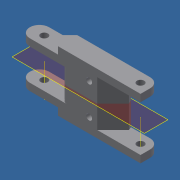
# Autodesk Inventor part: FingerPartA
Saved by Autodesk Inventor 2014 SP2 (Build 180246200, 246)
## iProperties
Created: 2014-12-28
Part Number: FingerPartA
Material: Generisch
Document SubType Name: Modeling
Designer: 4ndreas
Density: 1 g/cm^3
Appearance: Vorgabe
Mass: 4.96399 g
Surface Area: 30.3488 cm^2
Volume: 4.96399 cm^3
Author: 4ndreas
Autodesk Inventor part; units mm, degrees
ref_plane "YZ Plane" through (0, 0, 0) normal (1, 0, 0) x (0, 1, 0)
ref_plane "XZ Plane" through (0, 0, 0) normal (0, 1, 0) x (-1, 0, 0)
ref_plane "XY Plane" through (0, 0, 0) normal (0, 0, 1) x (1, 0, 0)
sketch "Skizze1" plane through (0, 0, 0) normal (0, 0, 1) x (1, 0, 0)
  circle A0 centre (0, 0) radius 4 construction
  circle A1 centre (40, 0) radius 4 construction
  line L0 (0, 0) -> (40, 0) construction
  arc A2 (0, 4) -> (0, -4) centre (0, 0) ccw
  arc A3 (44, 0) -> (40, 4) centre (40, 0) ccw
  line L1 (0, 4) -> (40, 4)
  line L2 (0, -4) -> (44, -4)
  line L3 (44, -4) -> (44, 0)
  dimension "d0" = 8
  dimension "d1" = 40
  constraints: 8 end point, 6 tangent, 4 centre point, 4 point on circle, 2 coincident, 1 equal radius, 1 horizontal, 1 parallel, 1 perpendicular
  measures "d0" diameter of A0
  measures "d1" distance of L0.start L0.end
extrude "Extrusion1" add sketch "Skizze1" along normal blind 3
sketch "Skizze2" plane through (0, 0, 3) normal (0, 0, 1) x (1, 0, 0)
  arc A0 (0, 4) -> (0, -4) centre (0, 0) ccw projected
  line L0 (0, -4) -> (44, -4) projected
  line L1 (44, -4) -> (44, 0) projected
  arc A1 (44, 0) -> (40, 4) centre (40, 0) ccw projected
  line L2 (40, 4) -> (0, 4) projected
  line L3 (6, 4) -> (34, 4)
  line L4 (34, 4) -> (34, -4)
  line L5 (34, -4) -> (6, -4)
  line L6 (6, -4) -> (6, 4)
  line L7 (0, 0) -> (-4, 0) construction
  line L8 (-4, 0) -> (-4, -4) construction
  line L9 (-4, -4) -> (0, -4) construction
  line L10 (0, -4) -> (0, 0) construction
  dimension "d4" = 10
  dimension "d5" = 4
  dimension "d6" = 10
  constraints: 16 end point, 4 parallel, 2 horizontal, 2 perpendicular, 2 point on line, 2 tangent
  measures "d4" distance between parallel lines of L4 L1
  measures "d5" radius of A1
  measures "d6" distance between parallel lines of L8 L6
extrude "Extrusion2" add sketch "Skizze2" along normal blind 9.5 contours L2 L4 L0 L6
sketch "Skizze3" plane through (0, 0, 0) normal (0, 0, -1) x (-1, 0, 0)
  line L0 (-6, -4) -> (-6, 4) projected
  line L1 (-6, 4) -> (0, 4) projected
  arc A0 (0, -4) -> (0, 4) centre (0, 0) ccw projected
  line L2 (0, -4) -> (-6, -4) projected
sketch "Skizze4" plane through (0, 0, 3) normal (0, 0, 1) x (1, 0, 0)
  line L0 (6, -4) -> (6, 4) projected
  line L1 (6, 4) -> (0, 4) projected
  arc A0 (0, 4) -> (0, -4) centre (0, 0) ccw projected
  line L2 (0, -4) -> (6, -4) projected
extrude "Extrusion3" add sketch "Skizze4" along normal blind 3
extrude "Extrusion4" cut sketch "Skizze3" against normal blind 3
sketch "Skizze5" plane through (0, 0, 0) normal (0, 0, -1) x (-1, 0, 0)
  line L0 (-6, -4) -> (-6, 4) projected
  line L1 (-40, 4) -> (-6, 4) projected
  arc A0 (-40, 4) -> (-44, 0) centre (-40, 0) ccw projected
  line L2 (-6, -4) -> (-44, -4) projected
  line L3 (-6, 0.3) -> (-9.7, 4)
  line L4 (-9.7, -4) -> (-6, -0.3)
  line L5 (-9.7, 4) -> (-6, 4)
  line L6 (-6, 0.3) -> (-6, 4)
  line L7 (0, 0) -> (-40, 0) construction
  circle A1 centre (0, 0) radius 4
  line L8 (-6, -4) -> (-6, 4) projected
  line L9 (0, -4) -> (-6, -4) projected
  arc A2 (0, -4) -> (0, 4) centre (0, 0) ccw projected
  line L10 (-6, 4) -> (0, 4) projected
  line L11 (-3.0018, 2.6437) -> (3.0018, -2.6437)
  line L12 (3.0018, -2.6437) -> (-9.9619, -17.3635)
  line L13 (-9.9619, -17.3635) -> (-15.9655, -12.0761)
  line L14 (-15.9655, -12.0761) -> (-3.0018, 2.6437)
  dimension "d13" = 45
  dimension "d14" = 0.6
  constraints: 18 end point, 6 point on line, 2 coincident, 2 parallel, 2 point on circle, 1 centre point, 1 collinear, 1 concentric, 1 midpoint, 1 perpendicular, 1 other
  measures "d13" angle of L3 L1
  measures "d14" distance of L3.start L4.end
extrude "Extrusion5" cut sketch "Skizze5" against normal up to surface (3 mm away) contours L0 L14 L2 L4 | L3 L1 L0 | L0 L2 L14
mirror "Spiegeln1" about plane through (20, 0, 12.5) normal (0, 0, 1)
sketch "Skizze6" plane through (6, -4, 19) normal (0, 0, -1) x (-1, 0, 0)
  line L0 (0, 8) -> (0, 0) projected
  line L1 (6, 0) -> (0, 0) projected
  arc A0 (6, 0) -> (6, 8) centre (6, 4) ccw projected
  line L2 (0, 8) -> (6, 8) projected
  line L3 (-3.7, 0) -> (-38, 0) projected
  line L4 (6, 0) -> (-3.7, 0) projected
  line L5 (0, 3.7) -> (-3.7, 0) projected
  line L6 (0, 3.7) -> (0, 4.3) projected
  line L7 (-3.7, 8) -> (0, 4.3) projected
  line L8 (-3.7, 8) -> (6, 8) projected
  arc A1 (6, 0) -> (6, 8) centre (6, 4) ccw projected
extrude "Extrusion6" cut sketch "Skizze6" along normal up to surface (13 mm away) contours L0 L7 L8 | L0 L4 L5
sketch "Skizze7" plane through (0, 0, 19) normal (0, 0, -1) x (-1, 0, 0)
  arc A0 (0, -4) -> (0, 4) centre (0, 0) ccw projected
  circle A1 centre (0, 0) radius 11.4
  circle A2 centre (0, 0) radius 13 construction
  dimension "d19" = 1.6
  dimension "d47" = 26
  constraints: 2 centre point, 2 coincident
  measures "d19" radial gap between concentric circles of A2 A1
  measures "d47" diameter of A2
extrude "Extrusion7" cut sketch "Skizze7" along normal up to surface (13 mm away)
sketch "Skizze8" plane through (44, -4, 22) normal (0, 0, -1) x (-1, 0, 0)
  line L0 (10, 8) -> (10, 0) projected
  line L1 (10, 0) -> (0, 0) projected
  line L2 (10, 8) -> (18, 0)
  line L3 (18, 0) -> (10, 0)
  point P0 (44, 4)
  dimension "d22" = 45
  constraints: 4 end point, 1 collinear
  measures "d22" angle of L0 L2
extrude "Extrusion8" cut sketch "Skizze8" along normal up to surface (19 mm away)
sketch "Skizze9" plane through (0, 0, 0) normal (0, 0, -1) x (-1, 0, 0)
  arc A0 (-40, 4) -> (-44, 0) centre (-40, 0) ccw projected
  point P0 (0, 0)
hole "Bohrung1" at (40, 0, 0) direction (0, 0, 1) diameter 3 end through all
hole "Bohrung2" at (0, 0, 0) direction (0, 0, 1) diameter 3 end through all
fillet "Rundung1" radius 2 2 edges at (10.6752, 4, 12.5) (10.6752, -4, 12.5)
chamfer "Fase1" distance 2 angle 45 1 edges at (34, 4, 12.5)
sketch "Skizze12" plane through (40, 4, 3) normal (0, 1, 0) x (1, 0, 0)
  line L0 (-8, 0) -> (-8, -19) projected
  line L1 (-26.7501, -3) -> (-8, -3)
  line L2 (-26.7501, -16) -> (-8, -16)
  point P0 (-40, 3)
  point P1 (-17.375, -3)
  point P2 (-17.375, -16)
  point P3 (-17.375, -3)
  point P4 (-17.375, -16)
  constraints: 4 end point, 2 coincident, 2 midpoint, 2 point on line, 1 parallel, 1 perpendicular
hole "Bohrung3" at (22.625, 4, 6) at (22.625, 4, 19) direction (0, -1, 0) diameter 2.5 end through all countersink diameter 4 countersink angle 90
sketch "Skizze13" plane through (0, -4, 22) normal (0, 0, 1) x (1, 0, 0)
  line L0 (0, 0) -> (9.7, 0) projected
  line L1 (9.7, 8) -> (0, 8) projected
  arc A0 (0, 8) -> (0, 0) centre (0, 4) ccw projected
  arc A1 (-2, 8) -> (-2, 0) centre (-2, 4) ccw
  line L2 (-2, 8) -> (0, 8)
  line L3 (0, 0) -> (-2, 0)
  dimension "d59" = 2
  constraints: 4 end point, 2 collinear, 2 point on circle, 2 tangent, 1 centre point
  measures "d59" distance of L2.start L1.end
extrude "Extrusion11" add sketch "Skizze13" against normal up to surface (3 mm away)
ref_plane "Arbeitsebene1" through (44, -4, 12.5) normal (0, 0, -1) x (-1, 0, 0)
mirror "Spiegeln2" about plane through (44, -4, 12.5) normal (0, 0, -1) of "Extrusion11"
equation "\"d0\" = Finger_diameter"
equation "\"d1\" = FingerLaenge_A"
equation "\"d2\" = FingerWall"
equation "\"d4\" = 2.5 * d5"
equation "\"d6\" = d4"
equation "\"d7\" = -0.5 * FingerWall + 0.5 * Finger_width"
equation "\"d9\" = FingerWall"
equation "\"d11\" = FingerWall"
equation "\"d15\" = FingerWall"
equation "\"d32\" = bearingHole"
equation "\"FingerLaenge_A\" = 40"
equation "\"FingerLaenge_B\" = 25"
equation "\"Hebel_B\" = 25"
equation "\"Finger_width\" = 22"
equation "\"Finger_diameter\" = 8"
equation "\"FingerWall\" = 3"
equation "\"Hebel_basis_2\" = 15"
equation "\"Join_width\" = 3"
equation "\"bearingHole\" = 3"
equation "\"bearingWall\" = 4"
equation "\"support_D\" = 0.25"
